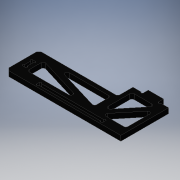
# Autodesk Inventor part: コックピット_2_メインフレーム_2
Saved by Autodesk Inventor 2018 (Build 220112000, 112)
## iProperties
Created: 2016-05-24
Part Number: コックピット_2_メインフレーム_2
Material: アセタール樹脂、黒
Document SubType Name: Modeling
Designer: hiroaki
Density: 1.425 g/cm^3
Appearance: 滑らか - 黒
Mass: 17.4619 g
Surface Area: 93.6545 cm^2
Volume: 12.254 cm^3
Author: hiroaki
Autodesk Inventor part; units mm, degrees
ref_plane "YZ Plane" through (0, 0, 0) normal (1, 0, 0) x (0, 1, 0)
ref_plane "XZ Plane" through (0, 0, 0) normal (0, 1, 0) x (-1, 0, 0)
ref_plane "XY Plane" through (0, 0, 0) normal (0, 0, 1) x (1, 0, 0)
derived "コックピット_2_基礎_2.ipt"
sketch "スケッチ1" plane through (0, 0, 0) normal (0, 0, 1) x (1, 0, 0)
  line L0 (-55, 16) -> (-55, -16) construction
  line L1 (-55, -16) -> (55, -16)
  line L2 (55, -16) -> (55, 31)
  line L3 (55, 31) -> (47.1, 31)
  line L4 (-55, 16) -> (20, 16)
  line L5 (20, 16) -> (20, 31)
  line L6 (20, 31) -> (27.9, 31)
  line L7 (30, 31) -> (30, 36)
  line L8 (30, 36) -> (45, 36)
  line L9 (45, 36) -> (45, 31)
  arc A0 (27.9, 31) -> (30, 31) centre (28.95, 31) ccw
  arc A1 (45, 31) -> (47.1, 31) centre (46.05, 31) ccw
  line L10 (37.5, 36) -> (37.5, -16) construction
  line L11 (-55, 16) -> (-50, 16) construction
  line L12 (-50, 16) -> (-50, -16) construction
  line L13 (-50, -16) -> (-55, -16) construction
  line L14 (-55, -16) -> (-55, 16) construction
  line L15 (-50, -16) -> (55, -16) construction
  line L16 (55, -16) -> (55, -11) construction
  line L17 (55, -11) -> (-50, -11) construction
  line L18 (-50, -11) -> (-50, -16) construction
  circle A2 centre (-52.5, 12) radius 1.55
  circle A3 centre (-52.5, -12) radius 1.55
  line L19 (-55, 0) -> (-50, 0) construction
  line L20 (-55, 16) -> (-57.5, 13.5)
  line L21 (-57.5, 13.5) -> (-57.5, -13.5)
  line L22 (-57.5, -13.5) -> (-55, -16)
  circle A4 centre (-52.5, 12) radius 3 construction
  line L23 (-50, 5) -> (-52.5, 5) construction
  line L24 (-52.5, 5) -> (-52.5, -5) construction
  line L25 (-52.5, -5) -> (-50, -5) construction
  line L26 (-50, -5) -> (-50, 5) construction
  line L27 (-30, -11) -> (35, -11) construction
  line L28 (35, -11) -> (35, -13.5) construction
  line L29 (35, -13.5) -> (-30, -13.5) construction
  line L30 (-30, -13.5) -> (-30, -11) construction
  line L31 (-52.55, -5.05) -> (-52.55, 5.05)
  line L32 (-52.55, 5.05) -> (-49.95, 5.05)
  line L33 (-49.95, 5.05) -> (-49.95, -5.05)
  line L34 (-49.95, -5.05) -> (-52.55, -5.05)
  circle A5 centre (-52.55, -4) radius 1.05
  circle A6 centre (-49.95, -4) radius 1.05
  circle A7 centre (-52.55, 4) radius 1.05
  circle A8 centre (-49.95, 4) radius 1.05
  line L35 (-30.05, -10.95) -> (35.05, -10.95)
  line L36 (35.05, -10.95) -> (35.05, -13.55)
  line L37 (35.05, -13.55) -> (-30.05, -13.55)
  line L38 (-30.05, -13.55) -> (-30.05, -10.95)
  circle A9 centre (-29, -13.55) radius 1.05
  circle A10 centre (-29, -10.95) radius 1.05
  circle A11 centre (34, -10.95) radius 1.05
  circle A12 centre (34, -13.55) radius 1.05
  point P0 (0, 0)
  point P1 (0, -16)
  point P2 (-52.5, 16)
  dimension "d13" = 2.1
  dimension "d14" = 0.05
  dimension "d15" = 0.05
  measures "d14" distance between parallel lines of L31 L24
  measures "d15" distance between parallel lines of L38 L30
extrude "押し出し1" add sketch "スケッチ1" along normal blind 5
sketch "スケッチ4" plane through (-55, -16, 5) normal (0, 0, 1) x (1, 0, 0)
  line L0 (87.95, 2.45) -> (27.05, 2.45) projected
  arc A0 (24.95, 2.45) -> (27.05, 2.45) centre (26, 2.45) ccw projected
  line L1 (24.95, 2.45) -> (24.95, 5.05) projected
  arc A1 (27.05, 5.05) -> (24.95, 5.05) centre (26, 5.05) ccw projected
  line L2 (27.05, 5.05) -> (87.95, 5.05) projected
  arc A2 (90.05, 5.05) -> (87.95, 5.05) centre (89, 5.05) ccw projected
  line L3 (90.05, 5.05) -> (90.05, 2.45) projected
  arc A3 (87.95, 2.45) -> (90.05, 2.45) centre (89, 2.45) ccw projected
  line L4 (110, 0) -> (110, 47) projected
  line L5 (82.9, 47) -> (75, 47) projected
  line L6 (75, 47) -> (75, 32) projected
  line L7 (75, 32) -> (0, 32) projected
  line L8 (5.05, 18.95) -> (5.05, 13.05) projected
  arc A4 (5.05, 10.95) -> (5.05, 13.05) centre (5.05, 12) ccw projected
  line L9 (5.05, 10.95) -> (2.45, 10.95) projected
  arc A5 (2.45, 13.05) -> (2.45, 10.95) centre (2.45, 12) ccw projected
  line L10 (2.45, 13.05) -> (2.45, 18.95) projected
  arc A6 (2.45, 21.05) -> (2.45, 18.95) centre (2.45, 20) ccw projected
  line L11 (2.45, 21.05) -> (5.05, 21.05) projected
  arc A7 (5.05, 18.95) -> (5.05, 21.05) centre (5.05, 20) ccw projected
  line L12 (9, 28) -> (72, 28) construction
  line L13 (72, 28) -> (72, 9) construction
  line L14 (72, 9) -> (9, 9) construction
  line L15 (9, 9) -> (9, 28) construction
  line L16 (79, 42) -> (106, 42) construction
  line L17 (106, 42) -> (106, 9) construction
  line L18 (106, 9) -> (79, 9) construction
  line L19 (79, 9) -> (79, 42) construction
  line L20 (9, 28) -> (72, 9) construction
  line L21 (79, 9) -> (106, 42) construction
  line L22 (17.6583, 28) -> (72, 28)
  line L23 (72, 28) -> (72, 11.6112)
  line L24 (72, 11.6112) -> (17.6583, 28)
  line L25 (9, 25.3888) -> (9, 9)
  line L26 (9, 9) -> (63.3417, 9)
  line L27 (63.3417, 9) -> (9, 25.3888)
  line L28 (5.05, 21) -> (2.45, 21) construction
  arc A8 (2.45, 21) -> (2.5, 19.0013) centre (2.45, 20) ccw construction
  line L29 (2.5, 19.0013) -> (2.5, 12.9987) construction
  arc A9 (2.5, 12.9987) -> (2.45, 11) centre (2.45, 12) ccw construction
  line L30 (2.45, 11) -> (5.05, 11) construction
  arc A10 (5.05, 11) -> (5, 12.9987) centre (5.05, 12) ccw construction
  line L31 (5, 12.9987) -> (5, 19.0013) construction
  arc A11 (5, 19.0013) -> (5.05, 21) centre (5.05, 20) ccw construction
  line L32 (88.0013, 5) -> (26.9987, 5) construction
  arc A12 (26.9987, 5) -> (25, 5.05) centre (26, 5.05) ccw construction
  line L33 (25, 5.05) -> (25, 2.45) construction
  arc A13 (25, 2.45) -> (26.9987, 2.5) centre (26, 2.45) ccw construction
  line L34 (26.9987, 2.5) -> (88.0013, 2.5) construction
  arc A14 (88.0013, 2.5) -> (90, 2.45) centre (89, 2.45) ccw construction
  line L35 (90, 2.45) -> (90, 5.05) construction
  arc A15 (90, 5.05) -> (88.0013, 5) centre (89, 5.05) ccw construction
  line L36 (79, 42) -> (102.7698, 42)
  line L37 (102.7698, 42) -> (79, 12.948)
  line L38 (79, 12.948) -> (79, 42)
  line L39 (82.2302, 9) -> (106, 9)
  line L40 (106, 9) -> (106, 38.052)
  line L41 (106, 38.052) -> (82.2302, 9)
  point P0 (55, 16)
  dimension "d16" = 0.05
  dimension "d17" = 4
  dimension "d18" = 4
  dimension "d19" = 0.05
  dimension "d20" = 4
  dimension "d21" = 5
  dimension "d22" = 3
  dimension "d23" = 4
  dimension "d24" = 4
  dimension "d25" = 5
  dimension "d26" = 5
  constraints: 60 end point, 16 point on circle, 9 collinear, 8 centre point, 8 parallel, 5 horizontal, 5 perpendicular, 1 point on line, 1 vertical, 16 other
  measures "d16" distance between parallel lines of L8 L31
  measures "d17" distance between parallel lines of L15 L31
  measures "d18" distance between parallel lines of L7 L12
  measures "d19" distance between parallel lines of L2 L32
  measures "d20" distance between parallel lines of L14 L32
  measures "d21" distance between parallel lines of L27 L24
  measures "d22" distance between parallel lines of L6 L13
  measures "d23" distance between parallel lines of L19 L6
  measures "d24" distance between parallel lines of L4 L17
  measures "d25" distance between parallel lines of L16 L5
  measures "d26" distance between parallel lines of L41 L37
extrude "押し出し2" cut sketch "スケッチ4" against normal blind 10 contours L22 L23 L24 | L27 L26 L25 | L36 L37 L38 | L41 L40 L39
fillet "フィレット1" radius 2 13 edges at (-37.3417, 12, 2.5) (8.3417, -7, 2.5) (17, -4.3888, 2.5) (24, -3.052, 2.5) (27.2302, -7, 2.5) (-46, -7, 2.5) (51, -7, 2.5) (47.7698, 26, 2.5) (51, 22.052, 2.5) (24, 26, 2.5) (17, 12, 2.5) (-46, 9.3888, 2.5) (20, 16, 2.5)
sketch "スケッチ6" plane through (55, -16, 0) normal (0, 0, -1) x (-1, 0, 0)
  circle A0 centre (107.5, 28) radius 1.55 projected
  circle A1 centre (107.5, 28) radius 1.55
  circle A2 centre (107.5, 4) radius 1.55 projected
  circle A3 centre (107.5, 4) radius 1.55
  point P0 (55, 16)
  constraints: 2 centre point, 2 coincident
extrude "押し出し3" add sketch "スケッチ6" against normal up to surface (5 mm away)
equation "\"d20\" = d17"
equation "\"d23\" = d18"
equation "\"d24\" = d18"
